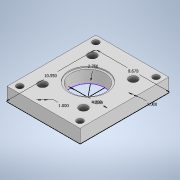
# Autodesk Inventor part: Wash_Base_Middle
Saved by Autodesk Inventor 2022 (Build 260153000, 153)
## iProperties
Created: 2021-10-22
Part Number: Wash_Base_Middle
Material: Generic
Document SubType Name: Modeling
Designer: tgr41
Density: 1 g/cm^3
Appearance: Default
Author: tgr41
Autodesk Inventor part; units mm, degrees
ref_plane "YZ Plane" through (0, 0, 0) normal (1, 0, 0) x (0, 1, 0)
ref_plane "XZ Plane" through (0, 0, 0) normal (0, 1, 0) x (-1, 0, 0)
ref_plane "XY Plane" through (0, 0, 0) normal (0, 0, 1) x (1, 0, 0)
sketch "Sketch1" plane through (0, 0, 0) normal (0, 1, 0) x (-1, 0, 0)
  line L0 (0, 0) -> (220.218, 0)
  line L1 (220.218, 0) -> (220.218, -267.97)
  line L2 (220.218, -267.97) -> (0, -267.97)
  line L3 (0, -267.97) -> (0, 0)
  circle A0 centre (110.109, -133.985) radius 57.15
  circle A1 centre (110.109, -133.985) radius 50.8
  line L4 (220.218, 0) -> (220.218, -25.4)
  line L5 (220.218, -133.985) -> (0, -133.985)
  line L6 (110.109, 0) -> (110.109, -267.97)
  line L7 (0, 0) -> (220.218, -267.97)
  line L8 (220.218, 0) -> (0, -267.97)
  line L9 (189.915, -36.8739) -> (146.3942, -89.8318)
  line L10 (220.218, -133.985) -> (167.259, -133.985)
  circle A2 centre (201.168, -248.92) radius 9.525
  circle A3 centre (201.168, -19.05) radius 9.525
  circle A4 centre (19.05, -248.92) radius 9.525
  circle A5 centre (19.05, -19.05) radius 9.525
  circle A6 centre (171.8873, -209.1593) radius 34.925
  circle A7 centre (48.3307, -209.1593) radius 34.925
  circle A8 centre (171.8873, -58.8107) radius 34.925
  circle A9 centre (48.3307, -58.8107) radius 34.925
  circle A10 centre (171.8873, -58.8107) radius 12.7
  circle A11 centre (171.8873, -209.1593) radius 12.7
  circle A12 centre (48.3307, -209.1593) radius 12.7
  circle A13 centre (48.3307, -58.8107) radius 12.7
  dimension "d0" = 220.218
  dimension "d1" = 267.97
  dimension "d11" = 114.3
  dimension "d12" = 101.6
  dimension "d40" = 69.85
  dimension "d41" = 25.4
  dimension "d42" = 25.4
  constraints: 22 end point, 14 centre point, 5 coincident, 4 midpoint, 4 point on line, 3 symmetric about line, 2 parallel, 2 point on circle, 1 horizontal, 1 perpendicular, 3 other
  measures "d0" distance of L1.end L2.end
  measures "d1" distance of L0.end L1.end
  measures "d11" diameter of A0
  measures "d12" diameter of A1
  measures "d40" diameter of A6
  measures "d41" diameter of A10
  measures "d42" diameter of A12
extrude "Extrusion3" add sketch "Sketch1" along normal blind 40.64
extrude "Extrusion4" cut sketch "Sketch1" along normal blind 40.64 contours L6 L7 A1 | A1 L8 L6 | L5 L8 A1 | A1 L7 L5 | A1 L5 L8 | L7 A1 L6 | L5 A1 L7 | L6 A1 L8
sketch "Sketch3" plane through (0, 40.64, 0) normal (0, 1, 0) x (1, 0, 0)
  line L0 (0, 267.97) -> (-220.218, 267.97) projected
  line L1 (-220.218, 0) -> (0, 0) projected
  circle A0 centre (-110.109, 133.985) radius 57.15
  dimension "d21" = 114.3
  constraints: 1 centre point
  measures "d21" diameter of A0
extrude "Extrusion6" cut sketch "Sketch3" against normal blind 3.175
extrude "Extrusion8" cut sketch "Sketch1" along normal blind 87.3125 contours A5 L7 | L7 A5 | A3 L8 | L8 A3 | A4 L8 | L8 A4 | A2 L7 | L7 A2
extrude "Extrusion9" cut sketch "Sketch1" along normal blind 96.8375 contours A13 L7 | L7 A13 | A10 L8 | L8 A10 | A12 L8 | L8 A12 | A11 L7 | L7 A11
body "Solid3"
